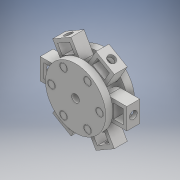
# Autodesk Inventor part: center-rotatry-mechanism
Saved by Autodesk Inventor 2018 (Build 220112000, 112)
## iProperties
Created: 2025-07-15
Part Number: center-rotatry-mechanism
Material: Generic
Document SubType Name: Modeling
Designer: neo
Density: 1 g/cm^3
Appearance: Default
Author: neo
Autodesk Inventor part; units mm, degrees
ref_plane "YZ Plane" through (0, 0, 0) normal (1, 0, 0) x (0, 1, 0)
ref_plane "XZ Plane" through (0, 0, 0) normal (0, 1, 0) x (-1, 0, 0)
ref_plane "XY Plane" through (0, 0, 0) normal (0, 0, 1) x (1, 0, 0)
sketch "Sketch1" plane through (0, 0, 0) normal (0, 1, 0) x (-1, 0, 0)
  circle A0 centre (0, 0) radius 1.6
  circle A1 centre (0, 0) radius 10 construction
  circle A2 centre (-10, 0) radius 1.6
  circle A3 centre (0, 0) radius 12.5
  dimension "d2" = 20
  dimension "d0" = 3.2
  dimension "d1" = 3.2
  dimension "d3" = 25
  constraints: 3 centre point, 3 coincident, 1 horizontal alignment, 2 other
  measures "d0" diameter of A0
  measures "d1" diameter of A2
  measures "d3" diameter of A3
extrude "Extrusion1" add sketch "Sketch1" along normal blind 3 contours A2 | A3
extrude "Extrusion2" cut sketch "Sketch1" along normal through all both and the other way through all contours A2
pattern_circular "Circular Pattern1" count 6 over 360 about axis through (0, 0, 0) along (0, 1, 0) of "Extrusion2"
sketch "Sketch2" plane through (0, 3, 0) normal (0, 1, 0) x (1, 0, 0)
  circle A0 centre (10, 0) radius 1.6 projected
  circle A1 centre (10, 0) radius 1.4
  arc A2 (10, 4.4) -> (10, -4.4) centre (10, 0) ccw
  line L0 (10, -4.4) -> (18, -4.4)
  line L1 (18, -4.4) -> (18, 4.4)
  line L2 (18, 4.4) -> (10, 4.4)
  line L3 (10, 1.6) -> (10, 1.4)
  line L4 (10, -1.4) -> (10, -1.6)
  point P0 (0, 0)
  dimension "d11" = 2.8
  dimension "d12" = 8.8
  dimension "d13" = 8
  constraints: 10 end point, 6 point on circle, 3 parallel, 2 centre point, 2 coincident, 1 horizontal, 1 perpendicular
  measures "d11" diameter of A1
  measures "d12" diameter of A2
  measures "d13" distance of L0.start L0.end
extrude "Extrusion3" add sketch "Sketch2" against normal up to surface (3 mm away) contours A1
extrude "Extrusion4" add sketch "Sketch2" along normal blind 3 contours A0 L4 A1 L3 | L3 A1 L4 A0 | A1 | L2 L1 L0 A2
sketch "Sketch3" plane through (0, 3, 0) normal (0, -1, 0) x (1, 0, 0)
  arc A0 (11.7, -4.4) -> (11.7, 4.4) centre (0, 0) ccw projected
  line L0 (11.7, -4.4) -> (18, -4.4) projected
  line L1 (18, -4.4) -> (18, 4.4) projected
  line L2 (18, 4.4) -> (11.7, 4.4) projected
  line L3 (10, -4.4) -> (11.7, -4.4) projected
  arc A1 (10, 4.4) -> (10, -4.4) centre (10, 0) ccw projected
  line L4 (11.7, 4.4) -> (10, 4.4) projected
  circle A2 centre (10, 0) radius 1.6 projected
  point P0 (0, 0)
extrude "Extrusion5" cut sketch "Sketch3" against normal blind 0.3
sketch "Sketch4" plane through (0, 6, 0) normal (0, 1, 0) x (1, 0, 0)
  arc A0 (10, 4.4) -> (10, -4.4) centre (10, 0) ccw projected
  line L0 (10, -4.4) -> (18, -4.4) projected
  line L1 (18, -4.4) -> (18, 4.4) projected
  line L2 (18, 4.4) -> (10, 4.4) projected
  line L3 (16.5, -2.9) -> (12.5, -2.9)
  line L4 (12.5, -2.9) -> (12.5, 2.9)
  line L5 (12.5, 2.9) -> (16.5, 2.9)
  line L6 (16.5, 2.9) -> (16.5, -2.9)
  point P0 (0, 0)
  dimension "d21" = 1.5
  dimension "d22" = 1.5
  dimension "d23" = 1.5
  dimension "d24" = 4
  constraints: 8 end point, 2 parallel, 1 horizontal, 1 perpendicular
  measures "d21" distance between parallel lines of L0 L3
  measures "d22" distance between parallel lines of L2 L5
  measures "d23" distance between parallel lines of L1 L6
  measures "d24" distance of L3.start L3.end
extrude "Extrusion6" cut sketch "Sketch4" against normal through all contours L3 L4 L5 L6
pattern_circular "Circular Pattern2" count 6 over 360 about axis through (0, 0, 0) along (0, 1, 0) of "Extrusion6", "Extrusion4", "Extrusion3", "Extrusion5"
mirror "Mirror1" about plane through (6.498, 6, 11.2548) normal (0, 1, 0)
sketch "Sketch5" plane through (18, 3.3, 4.4) normal (1, 0, 0) x (0, 0, -1)
  line L0 (0, 0) -> (8.8, 0) projected
  line L1 (8.8, 0) -> (8.8, 5.4) projected
  line L2 (0, 5.4) -> (8.8, 5.4) projected
  line L3 (0, 0) -> (0, 5.4) projected
  line L4 (0, 5.4) -> (8.8, 0)
  line L5 (8.8, 5.4) -> (0, 5.4) projected
  line L6 (8.8, 0) -> (0, 0) projected
  line L7 (8.8, 5.4) -> (0, 0)
  circle A0 centre (4.4, 2.7) radius 1.6
  point P0 (4.4, -3.3)
  dimension "d30" = 3.2
  constraints: 4 end point, 1 centre point, 1 midpoint
  measures "d30" diameter of A0
hole "Hole1" at (18, 6, 0) direction (-1, 0, 0) diameter 3.2 depth 3 tip angle 118
pattern_circular "Circular Pattern3" count 6 over 360 about axis through (0, 12, 0) along (0, 1, 0) of "Hole1"
sketch "Sketch6" plane through (0, 12, 0) normal (0, 1, 0) x (1, 0, 0)
  circle A0 centre (0, 0) radius 3.5
  circle A1 centre (0, 0) radius 1.6 projected
  dimension "d41" = 7
  constraints: 1 centre point, 1 coincident
  measures "d41" diameter of A0
extrude "Extrusion7" add sketch "Sketch6" against normal through all
body "Solid1"
